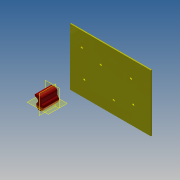
# Autodesk Inventor part: PunchBooleanExample
Saved by Autodesk Inventor 2015 (Build 190159000, 159)
## iProperties
Created: 2014-09-22
Part Number: PunchBooleanExample
Material: Generic
Document SubType Name: Modeling
Designer: ekinsb
Density: 1 g/cm^3
Appearance: Default
Author: Brian Ekins
Autodesk Inventor part; units mm, degrees
sketch "Sketch1" plane through (0, 0, 0) normal (0, 0, 1) x (1, 0, 0)
  line L0 (44.3308, 42.9963) -> (272.2828, 42.9963)
  line L1 (272.2828, 42.9963) -> (272.2828, 204.2861)
  line L2 (272.2828, 204.2861) -> (44.3308, 204.2861)
  line L3 (44.3308, 204.2861) -> (44.3308, 42.9963)
  point P0 (0, 0)
  constraints: 8 end point, 2 parallel, 1 horizontal, 1 perpendicular
extrude "Extrusion1" add sketch "Sketch1" along normal blind 3.175
sketch "Sketch2" plane through (0, 0, 0) normal (0, 0, 1) x (1, 0, 0)
  arc A0 (-6.2895, 7.9792) -> (6.2895, 7.9792) centre (0, 0) ccw
  line L0 (-5.08, 10.4727) -> (-5.08, 12.4251)
  arc A1 (-5.08, 12.4251) -> (-10.4349, 17.78) centre (-10.4349, 12.4251) ccw
  arc A2 (-10.4349, 25.4) -> (-10.4349, 17.78) centre (-10.4349, 21.59) ccw
  line L1 (-10.4349, 25.4) -> (-1.27, 25.4)
  arc A3 (5.08, 19.05) -> (-1.27, 25.4) centre (-1.27, 19.05) ccw
  line L2 (5.08, 19.05) -> (5.08, 10.4727)
  arc A4 (-6.2895, 7.9792) -> (-5.08, 10.4727) centre (-8.255, 10.4727) ccw
  arc A5 (5.08, 10.4727) -> (6.2895, 7.9792) centre (8.255, 10.4727) ccw
  point P0 (-5.08, 8.7988)
  point P1 (5.08, 8.7988)
  dimension "d4" = 3.175
  dimension "d5" = 10.16
  dimension "d6" = 3.81
  dimension "d7" = 5.3549
  dimension "d8" = 6.35
  dimension "d9" = 25.4
  dimension "d10" = 10.16
  dimension "d11" = 5.08
  constraints: 14 point on circle, 9 tangent, 6 centre point, 6 end point, 2 point on line, 1 coincident, 1 equal radius, 1 perpendicular, 1 vertical alignment, 1 other
  measures "d4" radius of A4
  measures "d5" radius of A0
  measures "d6" radius of A2
  measures "d7" radius of A1
  measures "d8" radius of A3
  measures "d9" distance from line of L1 point (0, 0)
  measures "d10" distance between parallel lines of L2 L0
  measures "d11" distance from line of L0 point (0, 0)
extrude "Extrusion2" add sketch "Sketch2" along normal blind 44.45 separate body
equation "\"d10\" = 2 * d11"
body "Solid1"
body "Solid2"
